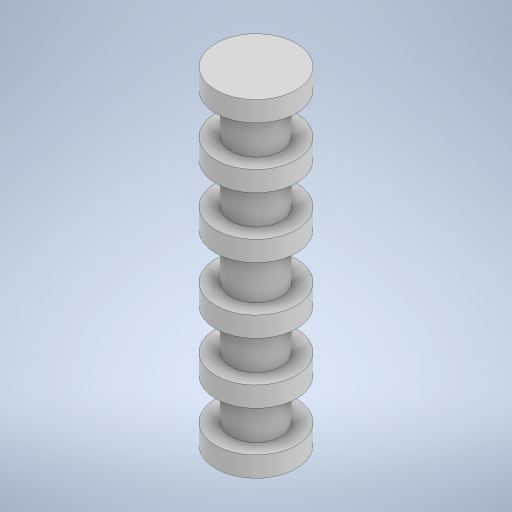
# Autodesk Inventor part: Crankshaft Crank Cylinder
Saved by Autodesk Inventor 2023 (Build 270158000, 158)
## iProperties
Created: 2022-10-29
Part Number: Crankshaft Crank Cylinder
Material: Generic
Document SubType Name: Modeling
Designer: tommy
Density: 1 g/cm^3
Appearance: Default
Author: tommy
Autodesk Inventor part; units mm, degrees
ref_plane "YZ Plane" through (0, 0, 0) normal (1, 0, 0) x (0, 1, 0)
ref_plane "XZ Plane" through (0, 0, 0) normal (0, 1, 0) x (-1, 0, 0)
ref_plane "XY Plane" through (0, 0, 0) normal (0, 0, 1) x (1, 0, 0)
sketch "Sketch1" plane through (0, 0, 0) normal (1, 0, 0) x (0, 1, 0)
  line L0 (0, 0) -> (0, -3.9878)
  line L1 (0, -3.9878) -> (0, -6.35)
  line L2 (0, -6.35) -> (3.175, -6.35)
  line L3 (3.175, -6.35) -> (3.175, -3.9878)
  line L4 (9.525, -3.9878) -> (9.525, -6.35)
  line L5 (9.525, -6.35) -> (12.7, -6.35)
  line L6 (12.7, -6.35) -> (12.7, -3.9878)
  line L7 (19.05, -3.9878) -> (19.05, -6.35)
  line L8 (19.05, -6.35) -> (22.225, -6.35)
  line L9 (22.225, -6.35) -> (22.225, -3.9878)
  line L10 (25.7937, 0) -> (0, 0)
  line L11 (51.5874, 0) -> (51.5874, -3.175)
  line L12 (51.5874, -3.175) -> (51.5874, -6.35)
  line L13 (51.5874, -6.35) -> (48.4124, -6.35)
  line L14 (48.4124, -6.35) -> (48.4124, -3.9878)
  line L15 (42.0624, -3.9878) -> (42.0624, -6.35)
  line L16 (42.0624, -6.35) -> (38.8874, -6.35)
  line L17 (38.8874, -6.35) -> (38.8874, -3.9878)
  line L18 (32.5374, -3.9878) -> (32.5374, -6.35)
  line L19 (32.5374, -6.35) -> (29.3624, -6.35)
  line L20 (29.3624, -6.35) -> (29.3624, -3.9878)
  line L21 (25.7937, 0) -> (51.5874, 0)
  line L22 (3.175, -3.9878) -> (9.525, -3.9878)
  line L23 (12.7, -3.9878) -> (19.05, -3.9878)
  line L24 (22.225, -3.9878) -> (29.3624, -3.9878)
  line L25 (32.5374, -3.9878) -> (38.8874, -3.9878)
  line L26 (42.0624, -3.9878) -> (48.4124, -3.9878)
  dimension "d1" = 3.9878
  dimension "d2" = 2.3622
  dimension "d3" = 3.175
  dimension "d5" = 3.175
  dimension "d7" = 3.175
  constraints: 54 end point, 10 perpendicular, 8 point on line, 1 vertical
  measures "d1" distance of L0.start L0.end
  measures "d2" distance of L0.end L1.end
  measures "d3" distance of L1.end L2.end
  measures "d5" distance of L4.end L5.end
  measures "d7" distance of L7.end L8.end
revolve "Revolution1" add sketch "Sketch1" angle 360 about axis through (0, 25.7937, 0) along (0, 1, 0)
body "Solid1"
